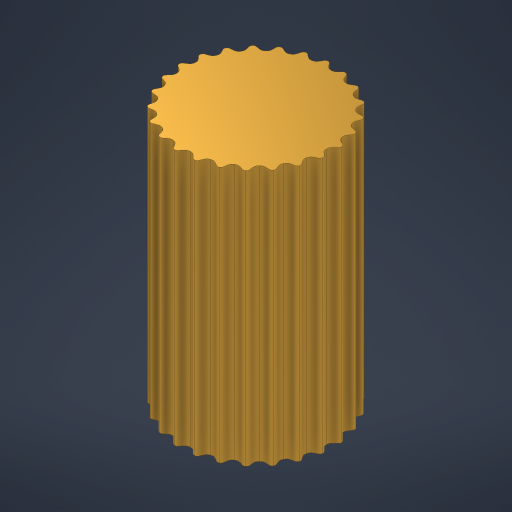
# Autodesk Inventor part: Zahnrad Servo
Saved by Autodesk Inventor 2023.2 (Build 272271000, 271)
## iProperties
Created: 2023-04-06
Part Number: Zahnrad Servo
Material: Messing, weicher Gelbton
Document SubType Name: Modeling
Designer: tadeus
Density: 8.47 g/cm^3
Appearance: Messing - satiniert
Author: tadeus
Autodesk Inventor part; units mm, degrees
ref_plane "YZ Plane" through (0, 0, 0) normal (1, 0, 0) x (0, 1, 0)
ref_plane "XZ Plane" through (0, 0, 0) normal (0, 1, 0) x (-1, 0, 0)
ref_plane "XY Plane" through (0, 0, 0) normal (0, 0, 1) x (1, 0, 0)
sketch "Skizze1" plane through (0, 0, 0) normal (0, 1, 0) x (-1, 0, 0)
  circle A0 centre (0, 0) radius 3 construction
  circle A1 centre (0, 0) radius 2.75 construction
  line L0 (2.75, 0) -> (3, 0) construction
  line L1 (2.7283, 0.3447) -> (2.9763, 0.376) construction
  line L2 (2.6636, 0.6839) -> (2.9057, 0.7461) construction
  line L3 (2.5569, 1.0123) -> (2.7893, 1.1044) construction
  line L4 (2.4098, 1.3248) -> (2.6289, 1.4453) construction
  line L5 (2.2248, 1.6164) -> (2.4271, 1.7634) construction
  line L6 (2.0047, 1.8825) -> (2.1869, 2.0536) construction
  line L7 (1.7529, 2.1189) -> (1.9123, 2.3115) construction
  line L8 (1.4735, 2.3219) -> (1.6075, 2.533) construction
  line L9 (1.1709, 2.4883) -> (1.2773, 2.7145) construction
  line L10 (0.8498, 2.6154) -> (0.9271, 2.8532) construction
  line L11 (0.5153, 2.7013) -> (0.5621, 2.9469) construction
  line L12 (0.1727, 2.7446) -> (0.1884, 2.9941) construction
  line L13 (-0.1727, 2.7446) -> (-0.1884, 2.9941) construction
  line L14 (-0.5153, 2.7013) -> (-0.5621, 2.9469) construction
  line L15 (-0.8498, 2.6154) -> (-0.9271, 2.8532) construction
  line L16 (-1.1709, 2.4883) -> (-1.2773, 2.7145) construction
  line L17 (-1.4735, 2.3219) -> (-1.6075, 2.533) construction
  line L18 (-1.7529, 2.1189) -> (-1.9123, 2.3115) construction
  line L19 (-2.0047, 1.8825) -> (-2.1869, 2.0536) construction
  line L20 (-2.2248, 1.6164) -> (-2.4271, 1.7634) construction
  line L21 (-2.4098, 1.3248) -> (-2.6289, 1.4453) construction
  line L22 (-2.5569, 1.0123) -> (-2.7893, 1.1044) construction
  line L23 (-2.6636, 0.6839) -> (-2.9057, 0.7461) construction
  line L24 (-2.7283, 0.3447) -> (-2.9763, 0.376) construction
  line L25 (-2.75, 0) -> (-3, 0) construction
  line L26 (-2.7283, -0.3447) -> (-2.9763, -0.376) construction
  line L27 (-2.6636, -0.6839) -> (-2.9057, -0.7461) construction
  line L28 (-2.5569, -1.0123) -> (-2.7893, -1.1044) construction
  line L29 (-2.4098, -1.3248) -> (-2.6289, -1.4453) construction
  line L30 (-2.2248, -1.6164) -> (-2.4271, -1.7634) construction
  line L31 (-2.0047, -1.8825) -> (-2.1869, -2.0536) construction
  line L32 (-1.7529, -2.1189) -> (-1.9123, -2.3115) construction
  line L33 (-1.4735, -2.3219) -> (-1.6075, -2.533) construction
  line L34 (-1.1709, -2.4883) -> (-1.2773, -2.7145) construction
  line L35 (-0.8498, -2.6154) -> (-0.9271, -2.8532) construction
  line L36 (-0.5153, -2.7013) -> (-0.5621, -2.9469) construction
  line L37 (-0.1727, -2.7446) -> (-0.1884, -2.9941) construction
  line L38 (0.1727, -2.7446) -> (0.1884, -2.9941) construction
  line L39 (0.5153, -2.7013) -> (0.5621, -2.9469) construction
  line L40 (0.8498, -2.6154) -> (0.9271, -2.8532) construction
  line L41 (1.1709, -2.4883) -> (1.2773, -2.7145) construction
  line L42 (1.4735, -2.3219) -> (1.6075, -2.533) construction
  line L43 (1.7529, -2.1189) -> (1.9123, -2.3115) construction
  line L44 (2.0047, -1.8825) -> (2.1869, -2.0536) construction
  line L45 (2.2248, -1.6164) -> (2.4271, -1.7634) construction
  line L46 (2.4098, -1.3248) -> (2.6289, -1.4453) construction
  line L47 (2.5569, -1.0123) -> (2.7893, -1.1044) construction
  line L48 (2.6636, -0.6839) -> (2.9057, -0.7461) construction
  line L49 (2.7283, -0.3447) -> (2.9763, -0.376) construction
  line L50 (2.7342, -0.2947) -> (2.7283, -0.3447) construction
  spline S0 degree 3 poles (3, 0) (3, -0.162) (2.7567, -0.111) (2.7283, -0.3447) knots 0 0 0 0 1 1 1 1
  line L51 (2.7374, -0.2699) -> (2.7192, -0.4195) construction
  arc A2 (2.7407, -0.2864) -> (2.7264, -0.4042) centre (3.0615, -0.3852) ccw construction
  line L52 (3, 0.0502) -> (3, -0.0502) construction
  arc A3 (2.9952, -0.039) -> (2.9952, 0.039) centre (2.8382, 0) ccw construction
  spline S1 degree 3 poles (3, 0) (3, 0.162) (2.7567, 0.111) (2.7283, 0.3447) knots 0 0 0 0 1 1 1 1
  line L53 (2.7374, 0.2699) -> (2.7192, 0.4195) construction
  arc A4 (2.7264, 0.4042) -> (2.7407, 0.2864) centre (3.0615, 0.3852) ccw construction
  line L54 (3, -0.0502) -> (3, 0.0502) construction
  arc A5 (2.9952, -0.039) -> (2.9952, 0.039) centre (2.8382, 0) ccw construction
  spline S2 degree 3 poles (2.9057, 0.7461) (2.8655, 0.903) (2.6425, 0.7931) (2.5569, 1.0123) knots 0 0 0 0 1 1 1 1
  line L55 (2.5843, 0.9422) -> (2.5295, 1.0825) construction
  line L56 (2.9182, 0.6974) -> (2.8933, 0.7947) construction
  arc A6 (2.5402, 1.0695) -> (2.5834, 0.959) centre (2.8696, 1.1345) ccw construction
  arc A7 (2.9108, 0.7071) -> (2.8914, 0.7827) centre (2.749, 0.7058) ccw construction
  spline S3 degree 3 poles (2.9057, 0.7461) (2.946, 0.5892) (2.6977, 0.5781) (2.7283, 0.3447) knots 0 0 0 0 1 1 1 1
  line L57 (2.7185, 0.4194) -> (2.7381, 0.27) construction
  line L58 (2.8933, 0.7947) -> (2.9182, 0.6974) construction
  arc A8 (2.7258, 0.4042) -> (2.7413, 0.2865) centre (3.0612, 0.3883) ccw construction
  arc A9 (2.9108, 0.7071) -> (2.8914, 0.7827) centre (2.749, 0.7058) ccw construction
  spline S4 degree 3 poles (2.6289, 1.4453) (2.5509, 1.5872) (2.3623, 1.4253) (2.2248, 1.6164) knots 0 0 0 0 1 1 1 1
  line L59 (2.2688, 1.5552) -> (2.1808, 1.6776) construction
  line L60 (2.6531, 1.4012) -> (2.6047, 1.4893) construction
  arc A10 (2.1944, 1.6677) -> (2.2637, 1.5713) centre (2.4973, 1.8125) ccw construction
  arc A11 (2.6435, 1.4088) -> (2.606, 1.4771) centre (2.4871, 1.3673) ccw construction
  spline S5 degree 3 poles (2.6289, 1.4453) (2.707, 1.3033) (2.4692, 1.2308) (2.5569, 1.0123) knots 0 0 0 0 1 1 1 1
  line L61 (2.5288, 1.0823) -> (2.5849, 0.9424) construction
  line L62 (2.6047, 1.4893) -> (2.6531, 1.4012) construction
  arc A12 (2.5397, 1.0694) -> (2.5839, 0.9593) centre (2.8684, 1.1374) ccw construction
  arc A13 (2.6435, 1.4088) -> (2.606, 1.4771) centre (2.4871, 1.3673) ccw construction
  spline S6 degree 3 poles (2.1869, 2.0536) (2.076, 2.1717) (1.9336, 1.968) (1.7529, 2.1189) knots 0 0 0 0 1 1 1 1
  line L63 (1.8107, 2.0706) -> (1.6951, 2.1672) construction
  line L64 (2.2213, 2.017) -> (2.1525, 2.0903) construction
  arc A14 (1.7108, 2.161) -> (1.8018, 2.0849) centre (1.9681, 2.3766) ccw construction
  arc A15 (2.2101, 2.0219) -> (2.1567, 2.0788) centre (2.069, 1.9429) ccw construction
  spline S7 degree 3 poles (2.1869, 2.0536) (2.2978, 1.9356) (2.0855, 1.8062) (2.2248, 1.6164) knots 0 0 0 0 1 1 1 1
  line L65 (2.1802, 1.6772) -> (2.2694, 1.5557) construction
  line L66 (2.1525, 2.0903) -> (2.2213, 2.017) construction
  arc A16 (2.194, 1.6674) -> (2.2642, 1.5717) centre (2.4954, 1.815) ccw construction
  arc A17 (2.2101, 2.0219) -> (2.1567, 2.0788) centre (2.069, 1.9429) ccw construction
  spline S8 degree 3 poles (1.6075, 2.533) (1.4707, 2.6198) (1.3834, 2.387) (1.1709, 2.4883) knots 0 0 0 0 1 1 1 1
  line L67 (1.2389, 2.4559) -> (1.1029, 2.5207) construction
  line L68 (1.6499, 2.5061) -> (1.5651, 2.5599) construction
  arc A18 (1.1196, 2.5186) -> (1.2267, 2.4675) centre (1.3152, 2.7913) ccw construction
  arc A19 (1.6379, 2.5081) -> (1.572, 2.5499) centre (1.5208, 2.3964) ccw construction
  spline S9 degree 3 poles (1.6075, 2.533) (1.7443, 2.4462) (1.5708, 2.2681) (1.7529, 2.1189) knots 0 0 0 0 1 1 1 1
  line L69 (1.6946, 2.1667) -> (1.8112, 2.0712) construction
  line L70 (1.5651, 2.5599) -> (1.6499, 2.5061) construction
  arc A20 (1.7104, 2.1606) -> (1.8022, 2.0854) centre (1.9657, 2.3786) ccw construction
  arc A21 (1.6379, 2.5081) -> (1.572, 2.5499) centre (1.5208, 2.3964) ccw construction
  spline S10 degree 3 poles (0.9271, 2.8532) (0.773, 2.9032) (0.7463, 2.6561) (0.5153, 2.7013) knots 0 0 0 0 1 1 1 1
  line L71 (0.5892, 2.6868) -> (0.4414, 2.7158) construction
  line L72 (0.9748, 2.8376) -> (0.8793, 2.8687) construction
  arc A22 (0.4581, 2.7179) -> (0.5745, 2.6951) centre (0.5797, 3.0307) ccw construction
  arc A23 (0.9627, 2.8366) -> (0.8885, 2.8607) centre (0.8771, 2.6993) ccw construction
  spline S11 degree 3 poles (0.9271, 2.8532) (1.0811, 2.8031) (0.9574, 2.5875) (1.1709, 2.4883) knots 0 0 0 0 1 1 1 1
  line L73 (1.1026, 2.52) -> (1.2392, 2.4565) construction
  line L74 (0.8793, 2.8687) -> (0.9748, 2.8376) construction
  arc A24 (1.1193, 2.5181) -> (1.2269, 2.4681) centre (1.3124, 2.7927) ccw construction
  arc A25 (0.9627, 2.8366) -> (0.8885, 2.8607) centre (0.8771, 2.6993) ccw construction
  spline S12 degree 3 poles (0.1884, 2.9941) (0.0267, 3.0043) (0.0623, 2.7583) (-0.1727, 2.7446) knots 0 0 0 0 1 1 1 1
  line L75 (-0.0975, 2.749) -> (-0.2479, 2.7402) construction
  line L76 (0.2385, 2.9909) -> (0.1382, 2.9972) construction
  arc A26 (-0.2322, 2.7464) -> (-0.1138, 2.7533) centre (-0.1922, 3.0797) ccw construction
  arc A27 (0.227, 2.9869) -> (0.1491, 2.9918) centre (0.1782, 2.8326) ccw construction
  spline S13 degree 3 poles (0.1884, 2.9941) (0.35, 2.9839) (0.2838, 2.7443) (0.5153, 2.7013) knots 0 0 0 0 1 1 1 1
  line L77 (0.4412, 2.7151) -> (0.5894, 2.6875) construction
  line L78 (0.1382, 2.9972) -> (0.2385, 2.9909) construction
  arc A28 (0.4579, 2.7173) -> (0.5746, 2.6956) centre (0.5767, 3.0313) ccw construction
  arc A29 (0.227, 2.9869) -> (0.1491, 2.9918) centre (0.1782, 2.8326) ccw construction
  spline S14 degree 3 poles (-0.5621, 2.9469) (-0.7213, 2.9165) (-0.6256, 2.6871) (-0.8498, 2.6154) knots 0 0 0 0 1 1 1 1
  line L79 (-0.778, 2.6384) -> (-0.9216, 2.5925) construction
  line L80 (-0.5128, 2.9563) -> (-0.6115, 2.9374) construction
  arc A30 (-0.9079, 2.6024) -> (-0.7949, 2.6385) centre (-0.952, 2.9351) ccw construction
  arc A31 (-0.5229, 2.9495) -> (-0.5996, 2.9349) centre (-0.5318, 2.7879) ccw construction
  spline S15 degree 3 poles (-0.5621, 2.9469) (-0.403, 2.9772) (-0.4076, 2.7287) (-0.1727, 2.7446) knots 0 0 0 0 1 1 1 1
  line L81 (-0.2478, 2.7395) -> (-0.0975, 2.7497) construction
  line L82 (-0.6115, 2.9374) -> (-0.5128, 2.9563) construction
  arc A32 (-0.2322, 2.7458) -> (-0.1138, 2.7538) centre (-0.1953, 3.0795) ccw construction
  arc A33 (-0.5229, 2.9495) -> (-0.5996, 2.9349) centre (-0.5318, 2.7879) ccw construction
  spline S16 degree 3 poles (-1.2773, 2.7145) (-1.4239, 2.6455) (-1.2742, 2.4471) (-1.4735, 2.3219) knots 0 0 0 0 1 1 1 1
  line L83 (-1.4097, 2.362) -> (-1.5373, 2.2818) construction
  line L84 (-1.2319, 2.7359) -> (-1.3228, 2.6931) construction
  arc A34 (-1.5266, 2.2948) -> (-1.4261, 2.3579) centre (-1.6521, 2.6062) ccw construction
  arc A35 (-1.24, 2.7268) -> (-1.3106, 2.6936) centre (-1.2084, 2.5681) ccw construction
  spline S17 degree 3 poles (-1.2773, 2.7145) (-1.1308, 2.7835) (-1.0734, 2.5416) (-0.8498, 2.6154) knots 0 0 0 0 1 1 1 1
  line L85 (-0.9213, 2.5918) -> (-0.7782, 2.639) construction
  line L86 (-1.3228, 2.6931) -> (-1.2319, 2.7359) construction
  arc A36 (-0.9078, 2.6018) -> (-0.7951, 2.639) centre (-0.955, 2.9342) ccw construction
  arc A37 (-1.24, 2.7268) -> (-1.3106, 2.6936) centre (-1.2084, 2.5681) ccw construction
  spline S18 degree 3 poles (-1.9123, 2.3115) (-2.0371, 2.2083) (-1.8427, 2.0534) (-2.0047, 1.8825) knots 0 0 0 0 1 1 1 1
  line L87 (-1.9528, 1.9372) -> (-2.0565, 1.8278) construction
  line L88 (-1.8736, 2.3436) -> (-1.951, 2.2795) construction
  arc A38 (-2.0493, 1.8431) -> (-1.9677, 1.9292) centre (-2.2483, 2.1134) ccw construction
  arc A39 (-1.8792, 2.3327) -> (-1.9393, 2.283) centre (-1.8091, 2.1869) ccw construction
  spline S19 degree 3 poles (-1.9123, 2.3115) (-1.7875, 2.4148) (-1.6717, 2.1948) (-1.4735, 2.3219) knots 0 0 0 0 1 1 1 1
  line L89 (-1.537, 2.2812) -> (-1.4101, 2.3626) construction
  line L90 (-1.951, 2.2795) -> (-1.8736, 2.3436) construction
  arc A40 (-1.5263, 2.2943) -> (-1.4264, 2.3584) centre (-1.6547, 2.6045) ccw construction
  arc A41 (-1.8792, 2.3327) -> (-1.9393, 2.283) centre (-1.8091, 2.1869) ccw construction
  spline S20 degree 3 poles (-2.4271, 1.7634) (-2.5223, 1.6323) (-2.2955, 1.5306) (-2.4098, 1.3248) knots 0 0 0 0 1 1 1 1
  line L91 (-2.3732, 1.3907) -> (-2.4464, 1.259) construction
  line L92 (-2.3975, 1.804) -> (-2.4566, 1.7227) construction
  arc A42 (-2.4433, 1.2755) -> (-2.3856, 1.3792) centre (-2.7032, 1.4879) ccw construction
  arc A43 (-2.4003, 1.7921) -> (-2.4461, 1.729) centre (-2.2962, 1.6683) ccw construction
  spline S21 degree 3 poles (-2.4271, 1.7634) (-2.3318, 1.8944) (-2.165, 1.7101) (-2.0047, 1.8825) knots 0 0 0 0 1 1 1 1
  line L93 (-2.056, 1.8273) -> (-1.9533, 1.9377) construction
  line L94 (-2.4566, 1.7227) -> (-2.3975, 1.804) construction
  arc A44 (-2.0489, 1.8427) -> (-1.9681, 1.9295) centre (-2.2504, 2.1112) ccw construction
  arc A45 (-2.4003, 1.7921) -> (-2.4461, 1.729) centre (-2.2962, 1.6683) ccw construction
  spline S22 degree 3 poles (-2.7893, 1.1044) (-2.849, 0.9538) (-2.604, 0.9116) (-2.6636, 0.6839) knots 0 0 0 0 1 1 1 1
  line L95 (-2.6445, 0.7568) -> (-2.6827, 0.611) construction
  line L96 (-2.7708, 1.1511) -> (-2.8078, 1.0577) construction
  arc A46 (-2.6837, 0.6278) -> (-2.6537, 0.7426) centre (-2.9884, 0.7689) ccw construction
  arc A47 (-2.7705, 1.1389) -> (-2.7993, 1.0664) centre (-2.6389, 1.0448) ccw construction
  spline S23 degree 3 poles (-2.7893, 1.1044) (-2.7297, 1.255) (-2.5223, 1.118) (-2.4098, 1.3248) knots 0 0 0 0 1 1 1 1
  line L97 (-2.4458, 1.2586) -> (-2.3739, 1.391) construction
  line L98 (-2.8078, 1.0577) -> (-2.7708, 1.1511) construction
  arc A48 (-2.4428, 1.2752) -> (-2.3861, 1.3795) centre (-2.7048, 1.4852) ccw construction
  arc A49 (-2.7705, 1.1389) -> (-2.7993, 1.0664) centre (-2.6389, 1.0448) ccw construction
  spline S24 degree 3 poles (-2.9763, 0.376) (-2.9966, 0.2153) (-2.7489, 0.2354) (-2.75, 0) knots 0 0 0 0 1 1 1 1
  line L99 (-2.7496, 0.0753) -> (-2.7504, -0.0753) construction
  line L100 (-2.97, 0.4258) -> (-2.9826, 0.3262) construction
  arc A50 (-2.7556, -0.0593) -> (-2.755, 0.0594) centre (-3.0857, 0.0016) ccw construction
  arc A51 (-2.9667, 0.4141) -> (-2.9765, 0.3367) centre (-2.8158, 0.3557) ccw construction
  spline S25 degree 3 poles (-2.9763, 0.376) (-2.956, 0.5367) (-2.7211, 0.4556) (-2.6636, 0.6839) knots 0 0 0 0 1 1 1 1
  line L101 (-2.682, 0.6108) -> (-2.6452, 0.757) construction
  line L102 (-2.9826, 0.3262) -> (-2.97, 0.4258) construction
  arc A52 (-2.6832, 0.6277) -> (-2.6542, 0.7427) centre (-2.9891, 0.7659) ccw construction
  arc A53 (-2.9667, 0.4141) -> (-2.9765, 0.3367) centre (-2.8158, 0.3557) ccw construction
  spline S26 degree 3 poles (-2.9763, -0.376) (-2.956, -0.5367) (-2.7211, -0.4556) (-2.6636, -0.6839) knots 0 0 0 0 1 1 1 1
  line L103 (-2.682, -0.6108) -> (-2.6452, -0.757) construction
  line L104 (-2.9826, -0.3262) -> (-2.97, -0.4258) construction
  arc A54 (-2.6542, -0.7427) -> (-2.6832, -0.6277) centre (-2.9891, -0.7659) ccw construction
  arc A55 (-2.9765, -0.3367) -> (-2.9667, -0.4141) centre (-2.8158, -0.3557) ccw construction
  spline S27 degree 3 poles (-2.9763, -0.376) (-2.9966, -0.2153) (-2.7489, -0.2354) (-2.75, 0) knots 0 0 0 0 1 1 1 1
  line L105 (-2.7496, -0.0753) -> (-2.7504, 0.0753) construction
  line L106 (-2.97, -0.4258) -> (-2.9826, -0.3262) construction
  arc A56 (-2.755, -0.0594) -> (-2.7556, 0.0593) centre (-3.0857, -0.0016) ccw construction
  arc A57 (-2.9765, -0.3367) -> (-2.9667, -0.4141) centre (-2.8158, -0.3557) ccw construction
  spline S28 degree 3 poles (-2.7893, -1.1044) (-2.7297, -1.255) (-2.5223, -1.118) (-2.4098, -1.3248) knots 0 0 0 0 1 1 1 1
  line L107 (-2.4458, -1.2586) -> (-2.3739, -1.391) construction
  line L108 (-2.8078, -1.0577) -> (-2.7708, -1.1511) construction
  arc A58 (-2.3861, -1.3795) -> (-2.4428, -1.2752) centre (-2.7048, -1.4852) ccw construction
  arc A59 (-2.7993, -1.0664) -> (-2.7705, -1.1389) centre (-2.6389, -1.0448) ccw construction
  spline S29 degree 3 poles (-2.7893, -1.1044) (-2.849, -0.9538) (-2.604, -0.9116) (-2.6636, -0.6839) knots 0 0 0 0 1 1 1 1
  line L109 (-2.6445, -0.7568) -> (-2.6827, -0.611) construction
  line L110 (-2.7708, -1.1511) -> (-2.8078, -1.0577) construction
  arc A60 (-2.6537, -0.7426) -> (-2.6837, -0.6278) centre (-2.9884, -0.7689) ccw construction
  arc A61 (-2.7993, -1.0664) -> (-2.7705, -1.1389) centre (-2.6389, -1.0448) ccw construction
  spline S30 degree 3 poles (-2.4271, -1.7634) (-2.3318, -1.8944) (-2.165, -1.7101) (-2.0047, -1.8825) knots 0 0 0 0 1 1 1 1
  line L111 (-2.056, -1.8273) -> (-1.9533, -1.9377) construction
  line L112 (-2.4566, -1.7227) -> (-2.3975, -1.804) construction
  arc A62 (-1.9681, -1.9295) -> (-2.0489, -1.8427) centre (-2.2504, -2.1112) ccw construction
  arc A63 (-2.4461, -1.729) -> (-2.4003, -1.7921) centre (-2.2962, -1.6683) ccw construction
  spline S31 degree 3 poles (-2.4271, -1.7634) (-2.5223, -1.6323) (-2.2955, -1.5306) (-2.4098, -1.3248) knots 0 0 0 0 1 1 1 1
  line L113 (-2.3732, -1.3907) -> (-2.4464, -1.259) construction
  line L114 (-2.3975, -1.804) -> (-2.4566, -1.7227) construction
  arc A64 (-2.3856, -1.3792) -> (-2.4433, -1.2755) centre (-2.7032, -1.4879) ccw construction
  arc A65 (-2.4461, -1.729) -> (-2.4003, -1.7921) centre (-2.2962, -1.6683) ccw construction
  spline S32 degree 3 poles (-1.9123, -2.3115) (-1.7875, -2.4148) (-1.6717, -2.1948) (-1.4735, -2.3219) knots 0 0 0 0 1 1 1 1
  line L115 (-1.537, -2.2812) -> (-1.4101, -2.3626) construction
  line L116 (-1.951, -2.2795) -> (-1.8736, -2.3436) construction
  arc A66 (-1.4264, -2.3584) -> (-1.5263, -2.2943) centre (-1.6547, -2.6045) ccw construction
  arc A67 (-1.9393, -2.283) -> (-1.8792, -2.3327) centre (-1.8091, -2.1869) ccw construction
  spline S33 degree 3 poles (-1.9123, -2.3115) (-2.0371, -2.2083) (-1.8427, -2.0534) (-2.0047, -1.8825) knots 0 0 0 0 1 1 1 1
  line L117 (-1.9528, -1.9372) -> (-2.0565, -1.8278) construction
  line L118 (-1.8736, -2.3436) -> (-1.951, -2.2795) construction
  arc A68 (-1.9677, -1.9292) -> (-2.0493, -1.8431) centre (-2.2483, -2.1134) ccw construction
  arc A69 (-1.9393, -2.283) -> (-1.8792, -2.3327) centre (-1.8091, -2.1869) ccw construction
  spline S34 degree 3 poles (-1.2773, -2.7145) (-1.1308, -2.7835) (-1.0734, -2.5416) (-0.8498, -2.6154) knots 0 0 0 0 1 1 1 1
  line L119 (-0.9213, -2.5918) -> (-0.7782, -2.639) construction
  line L120 (-1.3228, -2.6931) -> (-1.2319, -2.7359) construction
  arc A70 (-0.7951, -2.639) -> (-0.9078, -2.6018) centre (-0.955, -2.9342) ccw construction
  arc A71 (-1.3106, -2.6936) -> (-1.24, -2.7268) centre (-1.2084, -2.5681) ccw construction
  spline S35 degree 3 poles (-1.2773, -2.7145) (-1.4239, -2.6455) (-1.2742, -2.4471) (-1.4735, -2.3219) knots 0 0 0 0 1 1 1 1
  line L121 (-1.4097, -2.362) -> (-1.5373, -2.2818) construction
  line L122 (-1.2319, -2.7359) -> (-1.3228, -2.6931) construction
  arc A72 (-1.4261, -2.3579) -> (-1.5266, -2.2948) centre (-1.6521, -2.6062) ccw construction
  arc A73 (-1.3106, -2.6936) -> (-1.24, -2.7268) centre (-1.2084, -2.5681) ccw construction
  spline S36 degree 3 poles (-0.5621, -2.9469) (-0.403, -2.9772) (-0.4076, -2.7287) (-0.1727, -2.7446) knots 0 0 0 0 1 1 1 1
  line L123 (-0.2478, -2.7395) -> (-0.0975, -2.7497) construction
  line L124 (-0.6115, -2.9374) -> (-0.5128, -2.9563) construction
  arc A74 (-0.1138, -2.7538) -> (-0.2322, -2.7458) centre (-0.1953, -3.0795) ccw construction
  arc A75 (-0.5996, -2.9349) -> (-0.5229, -2.9495) centre (-0.5318, -2.7879) ccw construction
  spline S37 degree 3 poles (-0.5621, -2.9469) (-0.7213, -2.9165) (-0.6256, -2.6871) (-0.8498, -2.6154) knots 0 0 0 0 1 1 1 1
  line L125 (-0.778, -2.6384) -> (-0.9216, -2.5925) construction
  line L126 (-0.5128, -2.9563) -> (-0.6115, -2.9374) construction
  arc A76 (-0.7949, -2.6385) -> (-0.9079, -2.6024) centre (-0.952, -2.9351) ccw construction
  arc A77 (-0.5996, -2.9349) -> (-0.5229, -2.9495) centre (-0.5318, -2.7879) ccw construction
  spline S38 degree 3 poles (0.1884, -2.9941) (0.35, -2.9839) (0.2838, -2.7443) (0.5153, -2.7013) knots 0 0 0 0 1 1 1 1
  line L127 (0.4412, -2.7151) -> (0.5894, -2.6875) construction
  line L128 (0.1382, -2.9972) -> (0.2385, -2.9909) construction
  arc A78 (0.5746, -2.6956) -> (0.4579, -2.7173) centre (0.5767, -3.0313) ccw construction
  arc A79 (0.1491, -2.9918) -> (0.227, -2.9869) centre (0.1782, -2.8326) ccw construction
  spline S39 degree 3 poles (0.1884, -2.9941) (0.0267, -3.0043) (0.0623, -2.7583) (-0.1727, -2.7446) knots 0 0 0 0 1 1 1 1
  line L129 (-0.0975, -2.749) -> (-0.2479, -2.7402) construction
  line L130 (0.2385, -2.9909) -> (0.1382, -2.9972) construction
  arc A80 (-0.1138, -2.7533) -> (-0.2322, -2.7464) centre (-0.1922, -3.0797) ccw construction
  arc A81 (0.1491, -2.9918) -> (0.227, -2.9869) centre (0.1782, -2.8326) ccw construction
  spline S40 degree 3 poles (0.9271, -2.8532) (1.0811, -2.8031) (0.9574, -2.5875) (1.1709, -2.4883) knots 0 0 0 0 1 1 1 1
  line L131 (1.1026, -2.52) -> (1.2392, -2.4565) construction
  line L132 (0.8793, -2.8687) -> (0.9748, -2.8376) construction
  arc A82 (1.2269, -2.4681) -> (1.1193, -2.5181) centre (1.3124, -2.7927) ccw construction
  arc A83 (0.8885, -2.8607) -> (0.9627, -2.8366) centre (0.8771, -2.6993) ccw construction
  spline S41 degree 3 poles (0.9271, -2.8532) (0.773, -2.9032) (0.7463, -2.6561) (0.5153, -2.7013) knots 0 0 0 0 1 1 1 1
  line L133 (0.5892, -2.6868) -> (0.4414, -2.7158) construction
  line L134 (0.9748, -2.8376) -> (0.8793, -2.8687) construction
  arc A84 (0.5745, -2.6951) -> (0.4581, -2.7179) centre (0.5797, -3.0307) ccw construction
  arc A85 (0.8885, -2.8607) -> (0.9627, -2.8366) centre (0.8771, -2.6993) ccw construction
  spline S42 degree 3 poles (1.6075, -2.533) (1.7443, -2.4462) (1.5708, -2.2681) (1.7529, -2.1189) knots 0 0 0 0 1 1 1 1
  line L135 (1.6946, -2.1667) -> (1.8112, -2.0712) construction
  line L136 (1.5651, -2.5599) -> (1.6499, -2.5061) construction
  arc A86 (1.8022, -2.0854) -> (1.7104, -2.1606) centre (1.9657, -2.3786) ccw construction
  arc A87 (1.572, -2.5499) -> (1.6379, -2.5081) centre (1.5208, -2.3964) ccw construction
  spline S43 degree 3 poles (1.6075, -2.533) (1.4707, -2.6198) (1.3834, -2.387) (1.1709, -2.4883) knots 0 0 0 0 1 1 1 1
  line L137 (1.2389, -2.4559) -> (1.1029, -2.5207) construction
  line L138 (1.6499, -2.5061) -> (1.5651, -2.5599) construction
  arc A88 (1.2267, -2.4675) -> (1.1196, -2.5186) centre (1.3152, -2.7913) ccw construction
  arc A89 (1.572, -2.5499) -> (1.6379, -2.5081) centre (1.5208, -2.3964) ccw construction
  spline S44 degree 3 poles (2.1869, -2.0536) (2.2978, -1.9356) (2.0855, -1.8062) (2.2248, -1.6164) knots 0 0 0 0 1 1 1 1
  line L139 (2.1802, -1.6772) -> (2.2694, -1.5557) construction
  line L140 (2.1525, -2.0903) -> (2.2213, -2.017) construction
  arc A90 (2.2642, -1.5717) -> (2.194, -1.6674) centre (2.4954, -1.815) ccw construction
  arc A91 (2.1567, -2.0788) -> (2.2101, -2.0219) centre (2.069, -1.9429) ccw construction
  spline S45 degree 3 poles (2.1869, -2.0536) (2.076, -2.1717) (1.9336, -1.968) (1.7529, -2.1189) knots 0 0 0 0 1 1 1 1
  line L141 (1.8107, -2.0706) -> (1.6951, -2.1672) construction
  line L142 (2.2213, -2.017) -> (2.1525, -2.0903) construction
  arc A92 (1.8018, -2.0849) -> (1.7108, -2.161) centre (1.9681, -2.3766) ccw construction
  arc A93 (2.1567, -2.0788) -> (2.2101, -2.0219) centre (2.069, -1.9429) ccw construction
  spline S46 degree 3 poles (2.6289, -1.4453) (2.707, -1.3033) (2.4692, -1.2308) (2.5569, -1.0123) knots 0 0 0 0 1 1 1 1
  line L143 (2.5288, -1.0823) -> (2.5849, -0.9424) construction
  line L144 (2.6047, -1.4893) -> (2.6531, -1.4012) construction
  arc A94 (2.5839, -0.9593) -> (2.5397, -1.0694) centre (2.8684, -1.1374) ccw construction
  arc A95 (2.606, -1.4771) -> (2.6435, -1.4088) centre (2.4871, -1.3673) ccw construction
  spline S47 degree 3 poles (2.6289, -1.4453) (2.5509, -1.5872) (2.3623, -1.4253) (2.2248, -1.6164) knots 0 0 0 0 1 1 1 1
  line L145 (2.2688, -1.5552) -> (2.1808, -1.6776) construction
  line L146 (2.6531, -1.4012) -> (2.6047, -1.4893) construction
  arc A96 (2.2637, -1.5713) -> (2.1944, -1.6677) centre (2.4973, -1.8125) ccw construction
  arc A97 (2.606, -1.4771) -> (2.6435, -1.4088) centre (2.4871, -1.3673) ccw construction
  spline S48 degree 3 poles (2.9057, -0.7461) (2.946, -0.5892) (2.6977, -0.5781) (2.7283, -0.3447) knots 0 0 0 0 1 1 1 1
  line L147 (2.7185, -0.4194) -> (2.7381, -0.27) construction
  line L148 (2.8933, -0.7947) -> (2.9182, -0.6974) construction
  arc A98 (2.7413, -0.2865) -> (2.7258, -0.4042) centre (3.0612, -0.3883) ccw construction
  arc A99 (2.8914, -0.7827) -> (2.9108, -0.7071) centre (2.749, -0.7058) ccw construction
  spline S49 degree 3 poles (2.9057, -0.7461) (2.8655, -0.903) (2.6425, -0.7931) (2.5569, -1.0123) knots 0 0 0 0 1 1 1 1
  line L149 (2.5843, -0.9422) -> (2.5295, -1.0825) construction
  line L150 (2.9182, -0.6974) -> (2.8933, -0.7947) construction
  arc A100 (2.5834, -0.959) -> (2.5402, -1.0695) centre (2.8696, -1.1345) ccw construction
  arc A101 (2.8914, -0.7827) -> (2.9108, -0.7071) centre (2.749, -0.7058) ccw construction
  point P0 (1.7529, 2.1189)
  point P1 (1.1709, 2.4883)
  point P2 (0.5153, 2.7013)
  point P3 (-0.1727, 2.7446)
  point P4 (-1.4735, 2.3219)
  point P5 (-2.0047, 1.8825)
  point P6 (-2.4098, 1.3248)
  point P7 (-2.6636, 0.6839)
  point P8 (-2.75, 0)
  point P9 (-2.6636, -0.6839)
  point P10 (-2.4098, -1.3248)
  point P11 (-1.4735, -2.3219)
  point P12 (-0.1727, -2.7446)
  point P13 (0.5153, -2.7013)
  point P14 (1.1709, -2.4883)
  point P15 (1.7529, -2.1189)
  point P16 (2.5569, -1.0123)
  point P17 (2.7283, -0.3447)
  point P18 (2.7283, 0.3447)
  dimension "d0" = 6
  dimension "d1" = 5.5
  dimension "d4" = 360
  dimension "d8" = 1
  dimension "d9" = 1.5
  dimension "d12" = 360
  constraints: 302 end point, 102 midpoint, 102 point on circle, 101 centre point, 9 symmetric about line, 3 vertical, 2 coincident, 2 horizontal, 1 horizontal alignment, 1158 other
  measures "d1" diameter of A1
extrude "Extrusion1" add sketch "Skizze1" along normal blind 10
